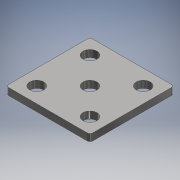
# Autodesk Inventor part: Piastra supporto pistone lama
Saved by Autodesk Inventor 2018 (Build 220112000, 112)
## iProperties
Created: 2020-06-15
Part Number: Piastra supporto pistone lama
Material: Generico
Document SubType Name: Modeling
Designer: Francesco
Density: 1 g/cm^3
Appearance: Acciaio - Lucido
Author: Francesco
Autodesk Inventor part; units mm, degrees
ref_plane "YZ Plane" through (0, 0, 0) normal (1, 0, 0) x (0, 1, 0)
ref_plane "XZ Plane" through (0, 0, 0) normal (0, 1, 0) x (-1, 0, 0)
ref_plane "XY Plane" through (0, 0, 0) normal (0, 0, 1) x (1, 0, 0)
sketch "Schizzo1" plane through (0, 0, 0) normal (0, 0, 1) x (1, 0, 0)
  line L0 (-30, 30) -> (30, 30)
  line L1 (30, 30) -> (30, -30)
  line L2 (30, -30) -> (-30, -30)
  line L3 (-30, -30) -> (-30, 30)
  line L4 (-30, 30) -> (30, -30) construction
  line L5 (30, 30) -> (-30, -30) construction
  circle A0 centre (0, 0) radius 5
  dimension "d0" = 60
  dimension "d1" = 60
  dimension "d5" = 10
  constraints: 12 end point, 2 midpoint, 2 parallel, 1 centre point, 1 coincident, 1 horizontal, 1 perpendicular
  measures "d0" distance of L1.end L2.end
  measures "d1" distance of L0.end L1.end
  measures "d5" diameter of A0
extrude "Estrusione2" add sketch "Schizzo1" along normal blind 5
fillet "Raccordo2" radius 5 4 edges at (-30, 30, 2.5) (30, 30, 2.5) (30, -30, 2.5) (-30, -30, 2.5)
sketch "Schizzo3" plane through (0, 0, 5) normal (0, 0, 1) x (1, 0, 0)
  circle A0 centre (19, -19) radius 6.4 projected
  circle A1 centre (-19, -19) radius 4.5 projected
  circle A2 centre (19, 19) radius 4.5 projected
  circle A3 centre (-19, 19) radius 3 projected
  point P0 (0, 0)
  constraints: 4 coincident
hole "Foro1" at (19, -19, 5) at (19, 19, 5) at (-19, 19, 5) at (-19, -19, 5) direction (0, 0, -1) diameter 10 end through all
